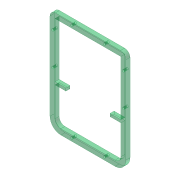
# Autodesk Inventor part: lcd_spacer
Saved by Autodesk Inventor 2014 (Build 180170000, 170)
## iProperties
Created: 2013-06-23
Part Number: lcd_spacer
Document SubType Name: Modeling
Designer: Administrator
Density: 1 g/cm^3
Material: Generic
Appearance: Clear - Green 1
Author: Administrator
Autodesk Inventor part; units mm, degrees
ref_plane "YZ Plane" through (0, 0, 0) normal (1, 0, 0) x (0, 1, 0)
ref_plane "XZ Plane" through (0, 0, 0) normal (0, 1, 0) x (-1, 0, 0)
ref_plane "XY Plane" through (0, 0, 0) normal (0, 0, 1) x (1, 0, 0)
sketch "Sketch1" plane through (0, 0, 0) normal (0, 0, 1) x (1, 0, 0)
  line L0 (11.7695, 33.9618) -> (11.7695, -67.6382)
  line L1 (100.6695, 33.9618) -> (100.6695, -67.6382)
  line L2 (18.1195, 40.3118) -> (94.3195, 40.3118)
  line L3 (24.4695, -80.3382) -> (87.9695, -80.3382)
  arc A0 (11.7695, -67.6382) -> (24.4695, -80.3382) centre (24.4695, -67.6382) ccw
  arc A1 (87.9695, -80.3382) -> (100.6695, -67.6382) centre (87.9695, -67.6382) ccw
  arc A2 (100.6695, 33.9618) -> (94.3195, 40.3118) centre (94.3195, 33.9618) ccw
  arc A3 (18.1195, 40.3118) -> (11.7695, 33.9618) centre (18.1195, 33.9618) ccw
  point P0 (0, 0)
  dimension "d0" = 12.7
  dimension "d1" = 6.35
  dimension "d2" = 120.65
  dimension "d3" = 88.9
  constraints: 8 end point, 8 point on circle, 8 tangent, 4 centre point, 2 equal radius, 2 horizontal, 2 vertical
  measures "d0" radius of A0
  measures "d1" radius of A3
  measures "d2" distance between parallel lines of L3 L2
  measures "d3" distance between parallel lines of L1 L0
extrude "Extrusion1" add sketch "Sketch1" along normal blind 4.7625
sketch "Sketch2" plane through (0, 0, 4.7625) normal (0, 0, 1) x (1, 0, 0)
  line L0 (11.7695, -67.6382) -> (11.7695, 33.9618) projected
  line L1 (100.6695, 33.9618) -> (100.6695, -67.6382) projected
  line L2 (18.1195, 40.3118) -> (94.3195, 40.3118) projected
  line L3 (17.7131, 34.3682) -> (94.7259, 34.3682)
  line L4 (94.7259, 34.3682) -> (94.7259, -29.6652)
  line L5 (94.7259, -29.6652) -> (17.7131, -29.6652)
  line L6 (17.7131, -29.6652) -> (17.7131, 34.3682)
  point P0 (0, 0)
  dimension "d6" = 5.9436
  dimension "d7" = 5.9436
  dimension "d8" = 5.9436
  dimension "d9" = 64.0334
  dimension "d54" = 77.0128
  constraints: 8 end point
  measures "d6" distance between parallel lines of L0 L6
  measures "d7" distance between parallel lines of L2 L3
  measures "d8" distance between parallel lines of L1 L4
  measures "d9" distance between parallel lines of L3 L5
  measures "d54" distance of L3.start L3.end
extrude "Extrusion2" cut sketch "Sketch2" against normal through all
sketch "Sketch3" plane through (0, 0, 4.7625) normal (0, 0, 1) x (1, 0, 0)
  line L0 (17.7131, -29.6652) -> (17.7131, 34.3682) projected
  line L1 (94.7259, 34.3682) -> (94.7259, -29.6652) projected
  line L2 (94.7259, -29.6652) -> (17.7131, -29.6652) projected
  line L3 (30.4131, -29.6652) -> (30.4131, -34.7452)
  line L4 (30.4131, -34.7452) -> (82.0259, -34.7452)
  line L5 (82.0259, -34.7452) -> (82.0259, -29.6652)
  point P0 (0, 0)
  dimension "d13" = 12.7
  dimension "d14" = 12.7
  dimension "d15" = 5.08
  constraints: 6 end point, 2 point on line
  measures "d13" distance between parallel lines of L0 L3
  measures "d14" distance between parallel lines of L1 L5
  measures "d15" distance between parallel lines of L2 L4
extrude "Extrusion3" cut sketch "Sketch3" against normal through all
sketch "Sketch4" plane through (0, 0, 4.7625) normal (0, 0, 1) x (1, 0, 0)
  line L0 (17.7131, -29.6652) -> (17.7131, 34.3682) projected
  line L1 (94.7259, 34.3682) -> (94.7259, -29.6652) projected
  line L2 (82.0259, -34.7452) -> (30.4131, -34.7452) projected
  arc A0 (11.7695, -67.6382) -> (24.4695, -80.3382) centre (24.4695, -67.6382) ccw projected
  line L3 (87.9695, -80.3382) -> (24.4695, -80.3382) projected
  arc A1 (87.9695, -80.3382) -> (100.6695, -67.6382) centre (87.9695, -67.6382) ccw projected
  line L4 (24.4695, -73.9882) -> (87.9695, -73.9882)
  line L5 (17.7131, -32.8402) -> (17.7131, -67.2318)
  line L6 (94.7259, -32.8402) -> (94.7259, -67.2318)
  arc A2 (17.7131, -67.2318) -> (24.4695, -73.9882) centre (24.4695, -67.2318) ccw
  arc A3 (87.9695, -73.9882) -> (94.7259, -67.2318) centre (87.9695, -67.2318) ccw
  line L7 (30.4131, -34.7452) -> (30.4131, -29.6652) projected
  line L8 (30.4131, -29.6652) -> (17.7131, -29.6652) projected
  line L9 (82.0259, -29.6652) -> (82.0259, -34.7452) projected
  line L10 (30.4131, -32.8402) -> (17.7131, -32.8402)
  line L11 (82.0259, -32.8402) -> (94.7259, -32.8402)
  point P0 (0, 0)
  dimension "d18" = 6.35
  dimension "d21" = 3.175
  constraints: 10 end point, 4 point on circle, 4 tangent, 3 collinear, 2 centre point, 2 horizontal, 2 point on line, 2 vertical alignment
  measures "d18" distance between parallel lines of L3 L4
  measures "d21" distance between parallel lines of L8 L10
extrude "Extrusion4" cut sketch "Sketch4" against normal through all
sketch "Sketch6" plane through (0, 0, 4.7625) normal (0, 0, 1) x (1, 0, 0)
  line L0 (87.9695, -80.3382) -> (24.4695, -80.3382) projected
  circle A0 centre (37.1695, 37.1876) radius 1.27
  circle A1 centre (75.2695, 37.1876) radius 1.27
  circle A2 centre (37.1695, -77.214) radius 1.27
  circle A3 centre (75.2695, -77.214) radius 1.27
  circle A4 centre (14.8937, 21.2618) radius 1.27
  circle A5 centre (14.8937, -16.8382) radius 1.27
  circle A6 centre (97.5453, 21.2618) radius 1.27
  circle A7 centre (97.5453, -16.8382) radius 1.27
  line L1 (18.1195, 40.3118) -> (94.3195, 40.3118) projected
  line L2 (11.7695, -67.6382) -> (11.7695, 33.9618) projected
  line L3 (100.6695, 33.9618) -> (100.6695, -67.6382) projected
  point P0 (0, 0)
  dimension "d35" = 3.1242
  dimension "d36" = 3.1242
  dimension "d37" = 3.1242
  dimension "d38" = 3.1242
  dimension "d39" = 2.54
  dimension "d40" = 25.4
  dimension "d41" = 19.05
  dimension "d42" = 25.4
  dimension "d43" = 38.1
  constraints: 8 centre point, 7 equal radius, 4 horizontal alignment, 4 vertical alignment
  measures "d35" distance from line of L0 A2.centre
  measures "d36" distance from line of L1 A0.centre
  measures "d37" distance from line of L2 A4.centre
  measures "d38" distance from line of L3 A6.centre
  measures "d39" diameter of A0
  measures "d40" distance from line of L2 A0.centre
  measures "d41" distance from line of L1 A4.centre
  measures "d42" distance from line of L3 A1.centre
  measures "d43" distance of A5.centre A4.centre
extrude "Extrusion5" cut sketch "Sketch6" against normal through all
sketch "Sketch7" plane through (0, 0, 4.7625) normal (0, 0, 1) x (1, 0, 0)
  circle A0 centre (97.5453, -16.8382) radius 1.27 projected
  circle A1 centre (97.5453, 21.2618) radius 1.27 projected
  circle A2 centre (14.8937, -16.8382) radius 1.27 projected
  circle A3 centre (14.8937, 21.2618) radius 1.27 projected
  circle A4 centre (75.2695, -77.214) radius 1.27 projected
  circle A5 centre (37.1695, -77.214) radius 1.27 projected
  circle A6 centre (75.2695, 37.1876) radius 1.27 projected
  circle A7 centre (37.1695, 37.1876) radius 1.27 projected
  line L0 (17.7131, -32.8402) -> (30.4131, -32.8402) projected
  line L1 (30.4131, -32.8402) -> (30.4131, -29.6652) projected
  line L2 (30.4131, -29.6652) -> (17.7131, -29.6652) projected
  line L3 (17.7131, -29.6652) -> (17.7131, 34.3682) projected
  line L4 (17.7131, 34.3682) -> (94.7259, 34.3682) projected
  line L5 (94.7259, 34.3682) -> (94.7259, -29.6652) projected
  line L6 (94.7259, -29.6652) -> (82.0259, -29.6652) projected
  line L7 (82.0259, -29.6652) -> (82.0259, -32.8402) projected
  line L8 (82.0259, -32.8402) -> (94.7259, -32.8402) projected
  line L9 (94.7259, -32.8402) -> (94.7259, -67.2318) projected
  arc A8 (87.9695, -73.9882) -> (94.7259, -67.2318) centre (87.9695, -67.2318) ccw projected
  line L10 (87.9695, -73.9882) -> (24.4695, -73.9882) projected
  arc A9 (17.7131, -67.2318) -> (24.4695, -73.9882) centre (24.4695, -67.2318) ccw projected
  line L11 (17.7131, -67.2318) -> (17.7131, -32.8402) projected
  arc A10 (18.1195, 40.3118) -> (11.7695, 33.9618) centre (18.1195, 33.9618) ccw projected
  line L12 (11.7695, -67.6382) -> (11.7695, 33.9618) projected
  arc A11 (11.7695, -67.6382) -> (24.4695, -80.3382) centre (24.4695, -67.6382) ccw projected
  line L13 (87.9695, -80.3382) -> (24.4695, -80.3382) projected
  arc A12 (87.9695, -80.3382) -> (100.6695, -67.6382) centre (87.9695, -67.6382) ccw projected
  line L14 (100.6695, 33.9618) -> (100.6695, -67.6382) projected
  arc A13 (100.6695, 33.9618) -> (94.3195, 40.3118) centre (94.3195, 33.9618) ccw projected
  line L15 (18.1195, 40.3118) -> (94.3195, 40.3118) projected
  line L16 (11.7695, -61.2882) -> (30.8195, -80.3382)
  line L17 (81.6195, -80.3382) -> (100.6695, -61.2882)
  point P0 (0, 0)
  dimension "d46" = 6.35
  dimension "d47" = 5.9436
  dimension "d48" = 82.9564
  dimension "d49" = 13.1064
  dimension "d50" = 12.7
  dimension "d51" = 19.05
  dimension "d52" = 19.05
  dimension "d53" = 69.85
  constraints: 8 point on line, 4 end point
  measures "d46" distance between parallel lines of L13 L10
  measures "d47" distance between parallel lines of L11 L12
  measures "d48" distance between parallel lines of L9 L12
  measures "d49" distance from line of L13 L11.start
  measures "d50" distance from line of L12 L10.end
  measures "d51" distance from line of L13 L16.start
  measures "d52" distance from line of L12 L16.end
  measures "d53" distance from line of L12 L17.start
body "Solid1"
